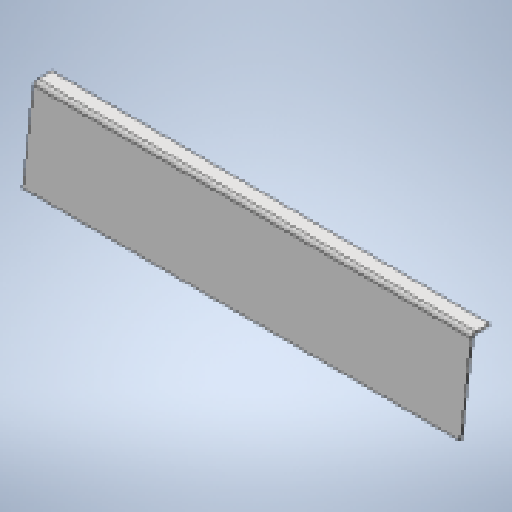
# Autodesk Inventor part: TRM 017 sheet in
Saved by Autodesk Inventor 2025 (Build 290162010, 162A)
## iProperties
Created: 2024-08-07
Part Number: TRM 017 sheet in
Material: AISI 304
Document SubType Name: Sheet Metal
Designer: pokla
Density: 8.02768 g/cm^3
Sheet Metal Rule: AISI304 2mm Die16
Sheet Metal Width: 0,000 mm
Sheet Metal Length: 0,000 mm
Sheet Metal Area: 0,000 mm^2
Appearance: Default
Stock Number: ТРМ 017 лист внутри
Author: pokla
Autodesk Inventor part; units mm, degrees
ref_plane "YZ Plane" through (0, 0, 0) normal (1, 0, 0) x (0, 1, 0)
ref_plane "XZ Plane" through (0, 0, 0) normal (0, 1, 0) x (-1, 0, 0)
ref_plane "XY Plane" through (0, 0, 0) normal (0, 0, 1) x (1, 0, 0)
sketch "Sketch7" plane through (0, 0, 0) normal (0, 0, 1) x (1, 0, 0)
  line L0 (250, 10) -> (-250, 10)
  line L1 (-250, 10) -> (-250, -10)
  line L2 (-250, -10) -> (250, -10)
  line L3 (250, -10) -> (250, 10)
  line L4 (250, 10) -> (-250, -10) construction
  line L5 (-250, 10) -> (250, -10) construction
  point P0 (0, 0)
  dimension "d52" = 500
  dimension "d53" = 20
  measures "d52" distance of L2.end L1.end
  measures "d53" distance of L1.end L0.end
extrude "Plate6" add sketch "Sketch7" along normal blind 2
sketch "Sketch8" plane through (-250, -8.0167, 1.7423) normal (0, -0.9916667, 0.1288302) x (1, 0, 0)
  line L0 (500, 0) -> (0, 0)
  line L1 (0, 0) -> (0, -100)
  line L2 (0, -100) -> (500, -100)
  line L3 (500, -100) -> (500, 0)
  constraints: 8 end point
edge flange "Flange5" height 100 angle 82.598 thickness 2 bend radius 2.75 thickness toward (0, -0.9916667, 0.1288302) relief round relief width 2 relief depth 1 edges at (0, -10, 0) wall of the first edge with corners at (250, -8.0167, 1.7423) (-250, -8.0167, 1.7423) (-250, -20.8997, -97.4243) (250, -20.8997, -97.4243)
bend "Bend5"
corner "Corner5"
equation "\"d54\" = Thickness"
equation "\"d55\" = BendReliefWidth"
equation "\"d56\" = BendReliefDepth"
equation "\"d57\" = MinimumRemnant"
equation "\"d58\" = TransitionRadius"
equation "\"d61\" = BendRadius"
equation "\"d62\" = CornerReliefSize"
equation "\"d63\" = GapSize"
equation "\"d64\" = JacobiRadiusSize"
equation "\"BendReliefWidth\" = Thickness"
equation "\"BendReliefDepth\" = 0.5 * Thickness"
equation "\"CornerReliefSize\" = 4 * Thickness"
equation "\"MinimumRemnant\" = 2 * Thickness"
equation "\"TransitionRadius\" = BendRadius"
equation "\"JacobiRadiusSize\" = BendRadius"
equation "\"GapSize\" = Thickness"
equation "\"Thickness\" = 2"
equation "\"BendRadius\" = 2.75"
body "Solid2"
